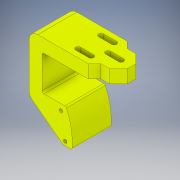
# Autodesk Inventor part: holder_outer
Saved by Autodesk Inventor 2019 (Build 230136000, 136)
## iProperties
Created: 2019-01-30
Part Number: holder_outer
Material: Generic
Document SubType Name: Modeling
Designer: suchanek
Density: 1 g/cm^3
Appearance: Default
Author: suchanek
Autodesk Inventor part; units mm, degrees
ref_plane "YZ Plane" through (0, 0, 0) normal (1, 0, 0) x (0, 1, 0)
ref_plane "XZ Plane" through (0, 0, 0) normal (0, 1, 0) x (-1, 0, 0)
ref_plane "XY Plane" through (0, 0, 0) normal (0, 0, 1) x (1, 0, 0)
sketch "Sketch1" plane through (0, 0, 0) normal (0, 0, 1) x (1, 0, 0)
  line L0 (-10, 0) -> (0, 0)
  line L1 (0, 0) -> (17.3648, -98.4808)
  line L2 (17.3648, -98.4808) -> (27.2129, -96.7443)
  line L3 (27.2129, -96.7443) -> (8.391, 10)
  line L4 (8.391, 10) -> (-10, 10)
  line L5 (-10, 10) -> (-10, 0)
  dimension "d0" = 80
  dimension "d1" = 10
  dimension "d2" = 10
  dimension "d3" = 10
  dimension "d4" = 100
  constraints: 12 end point, 4 perpendicular, 1 horizontal
  measures "d0" angle of L0 L1
  measures "d1" distance of L0.start L0.end
  measures "d2" distance between parallel lines of L4 L0
  measures "d3" distance between parallel lines of L1 L3
  measures "d4" distance of L0.end L1.end
sketch "Sketch2" plane through (0, 0, 0) normal (0, 0, 1) x (1, 0, 0)
  line L0 (18.1173, -67.6148) -> (56.6427, 18.898)
  line L1 (27.94, 25) -> (-20, 10)
  line L2 (0, 0) -> (-20, 0)
  line L3 (-20, 0) -> (-20, 10)
  line L4 (0, 0) -> (18.1173, -67.6148)
  line L5 (0, 0) -> (70, 0) construction
  circle A0 centre (42.94, 25) radius 15
  circle A1 centre (42.94, 25) radius 5
  line L6 (-20, 10) -> (25, 10)
  dimension "d5" = 20
  dimension "d6" = 10
  dimension "d7" = 70
  dimension "d8" = 75
  dimension "d9" = 30
  dimension "d10" = 10
  dimension "d61" = 62.94
  constraints: 14 end point, 3 horizontal, 2 centre point, 2 point on circle, 2 tangent, 1 coincident, 1 equal length, 1 horizontal alignment, 1 vertical
  measures "d5" distance of L2.start L2.end
  measures "d6" distance of L2.end L1.end
  measures "d7" distance of L2.start L0.start
  measures "d8" angle of L4 L5
  measures "d9" diameter of A0
  measures "d10" diameter of A1
  measures "d61" distance from line of A0.centre L3
extrude "Extrusion1" add sketch "Sketch1" along normal mid plane 100
extrude "Extrusion2" add sketch "Sketch2" along normal mid plane 30
sketch "Sketch3" plane through (0, 0, 15) normal (0, 0, 1) x (1, 0, 0)
  line L0 (20.9536, -61.2458) -> (8.391, 10) projected
  line L1 (56.6427, 10) -> (8.391, 10)
  arc A0 (56.6427, 18.898) -> (27.94, 25) centre (42.94, 25) ccw projected
  line L2 (57.94, 25) -> (57.94, -20)
  line L3 (57.94, -20) -> (13.6808, -20)
  line L4 (20.9536, -61.2458) -> (56.6427, 18.898) projected
  line L5 (56.6427, 10) -> (57.94, 10)
  point P0 (42.941, 25)
  point P1 (9.2838, 4.9367)
  point P2 (57.94, 10)
  dimension "d23" = 30
  constraints: 8 end point, 3 point on line, 2 perpendicular, 1 horizontal, 1 point on circle, 1 tangent, 1 vertical
  measures "d23" distance between parallel lines of L3 L1
extrude "Extrusion3" add sketch "Sketch3" against normal up to surface (100 mm away) from surface at 35 contours L0 L1 L4 L3 | L4 L1 L5 L2 L3 | L4 A0 L2 L5 L1
extrude "Extrusion5" add sketch "Sketch3" against normal up to surface (30 mm away)
sketch "Sketch5" plane through (57.94, 10, 15) normal (1, 0, 0) x (0, 0, -1)
  line L0 (65, -10) -> (-35, -10) projected
  line L1 (-23, -10) -> (-3, -10)
  line L2 (-3, -10) -> (-3, -20)
  line L3 (-3, -20) -> (-23, -20)
  line L4 (-23, -20) -> (-23, -10)
  line L5 (0, 0) -> (0, 15) projected
  line L6 (15, -10) -> (15, 0)
  line L7 (53, -10) -> (33, -10)
  line L8 (33, -10) -> (33, -20)
  line L9 (33, -20) -> (53, -20)
  line L10 (53, -20) -> (53, -10)
  dimension "d26" = 20
  dimension "d27" = 10
  dimension "d28" = 3
  constraints: 18 end point, 4 symmetric about line, 2 parallel, 1 horizontal, 1 perpendicular, 1 point on line, 1 vertical
  measures "d26" distance of L2.end L3.end
  measures "d27" distance of L1.end L2.end
  measures "d28" distance between parallel lines of L5 L2
extrude "Extrusion6" cut sketch "Sketch5" against normal blind 50
sketch "Sketch6" plane through (-10, 10, 50) normal (0, 1, 0) x (1, 0, 0)
  circle A0 centre (32.94, 22) radius 2.6
  line L0 (32.94, 22) -> (54.1621, 22)
  line L1 (67.94, 32) -> (17.94, 32) projected
  line L2 (67.94, 32) -> (72.1451, 32)
  line L3 (67.94, 12) -> (17.94, 12) projected
  line L4 (67.94, 12) -> (72.1451, 12)
  line L5 (67.94, 32) -> (70.0688, 32)
  line L6 (67.94, 12) -> (80.0698, 12)
  arc A1 (56.4323, 13.4495) -> (56.4323, 30.5505) centre (32.94, 22) ccw
  line L7 (32.94, 22) -> (56.4323, 13.4495) construction
  line L8 (32.94, 22) -> (57.94, 22) construction
  line L9 (32.94, 22) -> (56.4323, 30.5505) construction
  arc A2 (61.3187, 11.671) -> (61.3187, 32.329) centre (32.94, 22) ccw
  line L10 (32.94, 22) -> (61.3187, 11.671) construction
  line L11 (32.94, 22) -> (63.14, 22) construction
  line L12 (32.94, 22) -> (61.3187, 32.329) construction
  arc A3 (61.3187, 32.329) -> (56.4323, 30.5505) centre (58.8755, 31.4398) ccw
  arc A4 (56.4323, 13.4495) -> (61.3187, 11.671) centre (58.8755, 12.5602) ccw
  line L13 (67.94, 35) -> (67.94, 0) projected
  point P0 (10, 50)
  point P1 (77.941, 35)
  point P2 (77.941, 5)
  point P3 (77.941, 0)
  dimension "d31" = 5.2
  dimension "d35" = 25
  dimension "d36" = 20
  dimension "d37" = 40
  dimension "d38" = 30.2
  dimension "d39" = 20
  dimension "d40" = 40
  dimension "d41" = 35
  constraints: 22 end point, 12 point on circle, 5 centre point, 5 horizontal, 3 coincident, 2 equal length, 2 point on line, 2 tangent, 2 other
  measures "d31" diameter of A0
  measures "d35" radius of A1
  measures "d36" angle of L7 L8
  measures "d37" angle of L7 L9
  measures "d38" radius of A2
  measures "d39" angle of L10 L11
  measures "d40" angle of L10 L12
extrude "Extrusion7" cut sketch "Sketch6" against normal up to surface (30 mm away) contours A0 | A2 L3 A4 A1 A3 L1 | L1 A3 A2 | A2 A4 L3
sketch "Sketch8" plane through (-10, 10, 50) normal (0, 1, 0) x (1, 0, 0)
  circle A0 centre (68.8765, 31.4398) radius 4.6
  arc A1 (71.3197, 32.329) -> (66.4333, 30.5505) centre (68.8765, 31.4398) ccw projected
  point P0 (10, 50)
  dimension "d49" = 9.2
  constraints: 1 centre point, 1 concentric
  measures "d49" diameter of A0
extrude "Extrusion9" cut sketch "Sketch8" along normal through all
sketch "Sketch9" plane through (57.94, 10, 15) normal (1, 0, 0) x (0, 0, -1)
  line L0 (-31, -20) -> (5, -20)
  line L1 (5, -20) -> (5, -10)
  line L2 (5, -10) -> (-31, -10)
  line L3 (-31, -10) -> (-31, -20)
  line L4 (-3, -20) -> (-23, -20) projected
  line L5 (-23, -10) -> (-3, -10) projected
  line L6 (-3, -10) -> (-3, -20) projected
  line L7 (-23, -20) -> (-23, -10) projected
  point P0 (15, -10)
  dimension "d53" = 8
  dimension "d58" = 8
  constraints: 8 end point, 2 collinear, 2 parallel, 1 horizontal, 1 perpendicular
  measures "d53" distance between parallel lines of L1 L6
  measures "d58" distance between parallel lines of L7 L3
loft "Loft1" cut profiles "Sketch9" section 2 edges at (7.94, -5, 38) (7.94, -10, 28) (7.94, -5, 18) (7.94, 0, 28)
mirror "Mirror2" about plane through (0, 0, 0) normal (0, 0, 1) of "Extrusion7", "Extrusion9", "Loft1"
sketch "Sketch10" plane through (0, 0, -15) normal (0, 0, -1) x (-1, 0, 0)
  line L0 (-57.941, 10) -> (10, 10)
  line L1 (10, 10) -> (10, 40)
  line L2 (10, 40) -> (-57.941, 40)
  line L3 (-57.941, 40) -> (-57.941, 10)
  arc A0 (-27.94, 25) -> (-55.9636, 32.4421) centre (-42.94, 25) ccw projected
  point P0 (0, 0)
  constraints: 8 end point, 2 parallel, 1 horizontal, 1 perpendicular, 1 point on line, 1 tangent
extrude "Extrusion10" cut sketch "Sketch10" along normal through all both and the other way through all
sketch "Sketch11" plane through (13.6808, -20, 15) normal (0, -1, 0) x (1, 0, 0)
  circle A0 centre (9.2592, 13) radius 2.6 projected
  line L0 (6.8632, 8.85) -> (4.4672, 13)
  line L1 (4.4672, 13) -> (6.8632, 17.15)
  line L2 (6.8632, 17.15) -> (11.6552, 17.15)
  line L3 (11.6552, 17.15) -> (14.0512, 13)
  line L4 (14.0512, 13) -> (11.6552, 8.85)
  line L5 (11.6552, 8.85) -> (6.8632, 8.85)
  circle A1 centre (9.2592, -43) radius 2.6 projected
  line L6 (6.8632, -47.15) -> (4.4672, -43)
  line L7 (4.4672, -43) -> (6.8632, -38.85)
  line L8 (6.8632, -38.85) -> (11.6552, -38.85)
  line L9 (11.6552, -38.85) -> (14.0512, -43)
  line L10 (14.0512, -43) -> (11.6552, -47.15)
  line L11 (11.6552, -47.15) -> (6.8632, -47.15)
  point P0 (-13.6808, -15)
  point P1 (9.2592, 13)
  point P2 (9.2592, -43)
  point P3 (9.2592, 8.85)
  dimension "d62" = 8.3
  dimension "d63" = 8.3
  constraints: 24 end point, 2 coincident, 1 horizontal, 1 horizontal alignment, 1 midpoint, 26 other
  measures "d62" distance between parallel lines of L10 L7
  measures "d63" distance between parallel lines of L5 L2
extrude "Extrusion11" cut sketch "Sketch11" against normal blind 3
sketch "Sketch12" plane through (-10, 0, 50) normal (0, -1, 0) x (1, 0, 0)
  line L0 (14.396, -41) -> (12, -36.85)
  line L1 (12, -36.85) -> (14.396, -32.7)
  line L2 (14.396, -32.7) -> (19.188, -32.7)
  line L3 (19.188, -32.7) -> (21.584, -36.85)
  line L4 (21.584, -36.85) -> (19.188, -41)
  line L5 (19.188, -41) -> (14.396, -41)
  line L6 (19.188, -59) -> (21.584, -63.15)
  line L7 (21.584, -63.15) -> (19.188, -67.3)
  line L8 (19.188, -67.3) -> (14.396, -67.3)
  line L9 (14.396, -67.3) -> (12, -63.15)
  line L10 (12, -63.15) -> (14.396, -59)
  line L11 (14.396, -59) -> (19.188, -59)
  line L12 (10, -50) -> (9.9797, -50)
  line L13 (10, -100) -> (10, 0) projected
  line L14 (10, -54.6091) -> (9.2997, -54.6091)
  line L15 (14.396, -67.3) -> (14.396, -59)
  line L16 (14.396, -41) -> (14.396, -32.7)
  line L17 (14.396, -41) -> (10, -41)
  line L18 (10, -41) -> (10, -32.7)
  line L19 (10, -32.7) -> (14.396, -32.7)
  line L20 (14.396, -32.7) -> (14.396, -41)
  line L21 (14.396, -67.3) -> (10, -67.3)
  line L22 (10, -67.3) -> (10, -59)
  line L23 (10, -59) -> (14.396, -59)
  line L24 (14.396, -59) -> (14.396, -67.3)
  circle A0 centre (16.792, -63.15) radius 2.8
  circle A1 centre (16.792, -36.85) radius 2.8
  dimension "d66" = 8.3
  dimension "d67" = 8.3
  dimension "d68" = 9
  dimension "d99" = 2
  dimension "d102" = 5.6
  dimension "d103" = 5.6
  constraints: 48 end point, 4 horizontal, 4 parallel, 3 collinear, 3 vertical, 2 centre point, 2 coincident, 2 perpendicular, 1 point on line, 32 other
  measures "d66" distance between parallel lines of L11 L8
  measures "d67" distance between parallel lines of L2 L5
  measures "d68" distance between parallel lines of L12 L11
  measures "d102" diameter of A0
  measures "d103" diameter of A1
extrude "Extrusion12" cut sketch "Sketch12" along normal blind 6 contours L16 A1 L2 L3 L4 L5 | L0 L1 L16 A1 | A1 L16 | L16 A1 | L6 L7 L8 L15 A0 L11 | L15 A0 L9 L10 | A0 L15 | L15 A0
extrude "Extrusion15" cut sketch "Sketch12" along normal blind 6 contours L17 L13 L19 L1 L0 | L16 A1 L2 L3 L4 L5 | L16 A1 | L6 L7 L8 L15 A0 L11 | L15 A0 L9 L10 | L10 L9 L21 L13 L23 | A0 L15 | L15 A0 picked at (16.128, -36.85)
sketch "Sketch15" plane through (0, 0, 15) normal (0, 0, 1) x (1, 0, 0)
  line L0 (-20, 0) -> (-20, 10) projected
  line L1 (-10, 13.1289) -> (-20, 10) projected
  line L2 (-20, 0) -> (-10, 0)
  line L3 (-10, 0) -> (-10, 13.1289)
  line L4 (-10, 13.1289) -> (-20, 13.1289)
  line L5 (-20, 13.1289) -> (-20, 0)
  point P0 (0, 0)
  constraints: 8 end point, 2 parallel, 1 horizontal, 1 perpendicular
extrude "Extrusion17" cut sketch "Sketch15" against normal blind 100 contours L0 L1 L3 L2
sketch "Sketch17" plane through (-10, 10, 50) normal (0, 1, 0) x (1, 0, 0)
  line L0 (0, 0) -> (0, 100) projected
  line L1 (27.3648, 0) -> (27.3648, 100) projected
  line L2 (0, 72.2615) -> (27.3648, 72.2615)
  line L3 (27.3648, 72.2615) -> (27.3648, 27.7385)
  line L4 (27.3648, 27.7385) -> (0, 27.7385)
  line L5 (0, 27.7385) -> (0, 72.2615)
  circle A0 centre (32.94, 78) radius 2.6 projected
  circle A1 centre (32.94, 22) radius 2.6 projected
  line L6 (27.3648, 27.7385) -> (34.6263, 35)
  line L7 (34.6263, 35) -> (44.6263, 35)
  line L8 (44.6263, 35) -> (54.6263, 45)
  line L9 (54.6263, 45) -> (54.6263, 55)
  line L10 (54.6263, 55) -> (44.6263, 65)
  line L11 (44.6263, 65) -> (34.6263, 65)
  line L12 (34.6263, 65) -> (27.3648, 72.2615)
  point P0 (10, 50)
  dimension "d134" = 8
  dimension "d135" = 8
  dimension "d136" = 45
  dimension "d137" = 45
  dimension "d138" = 135
  dimension "d139" = 135
  dimension "d140" = 10
  dimension "d141" = 30
  constraints: 22 end point, 3 horizontal, 3 point on line, 2 equal length, 2 parallel, 1 perpendicular, 1 vertical
  measures "d134" distance from line of A0.centre L12
  measures "d135" distance from line of A1.centre L6
  measures "d136" angle of L3 L6
  measures "d137" angle of L3 L12
  measures "d138" angle of L11 L10
  measures "d139" angle of L8 L7
  measures "d140" distance of L8.end L9.end
  measures "d141" distance between parallel lines of L11 L7
extrude "Extrusion18" add sketch "Sketch17" along normal blind 15 contours L0 L2 L1 L4 | L1 L12 L11 L10 L9 L8 L7 L6
extrude "Extrusion16" cut sketch "Sketch12" against normal blind 100 and the other way blind 10 contours A1 L16 | L16 A1 | A0 L15 | L15 A0
sketch "Sketch13" plane through (-10, 10, 50) normal (0, 1, 0) x (1, 0, 0)
  line L0 (10, 50) -> (37.94, 50)
  line L1 (27.3648, 0) -> (27.3648, 100) projected
  circle A0 centre (37.94, 50) radius 2.8
  line L2 (67.94, 100) -> (67.94, 0) projected
  dimension "d85" = 5.6
  dimension "d108" = 30
  constraints: 2 end point, 1 centre point, 1 coincident, 1 horizontal
  measures "d85" diameter of A0
  measures "d108" distance from line of A0.centre L2
extrude "Extrusion13" cut sketch "Sketch13" against normal blind 30 and the other way blind 150
sketch "Sketch14" plane through (27.94, -20, 0) normal (0, 1, 0) x (1, 0, 0)
  line L0 (-10.5752, -50) -> (-10.5752, 50) projected
  line L1 (-2.4249, -4.2) -> (-4.8497, 0)
  line L2 (-4.8497, 0) -> (-2.4249, 4.2)
  line L3 (-2.4249, 4.2) -> (2.4249, 4.2)
  line L4 (2.4249, 4.2) -> (4.8497, 0)
  line L5 (4.8497, 0) -> (2.4249, -4.2)
  line L6 (2.4249, -4.2) -> (-2.4249, -4.2)
  circle A0 centre (0, 0) radius 2.8 projected
  line L7 (-2.4249, 4.2) -> (-32.4249, 4.2)
  line L8 (-32.4249, 4.2) -> (-32.4249, -4.2)
  line L9 (-32.4249, -4.2) -> (-2.4249, -4.2)
  line L10 (-2.4249, -4.2) -> (-2.4249, 4.2)
  point P0 (-27.94, 0)
  point P1 (-10.5752, -4.2)
  dimension "d88" = 8.4
  dimension "d89" = 30
  constraints: 20 end point, 2 coincident, 2 horizontal, 2 parallel, 1 collinear, 1 perpendicular, 1 point on line, 15 other
  measures "d88" distance between parallel lines of L3 L6
  measures "d89" distance of L2.end L7.end
hole "Hole3" at (27.94, -20, 0) direction (0, -1, 0) diameter 5.2 depth 5 tip angle 118
extrude "Extrusion14" cut sketch "Sketch14" along normal blind 6
sketch "Sketch18" plane through (-10, 10, 22.2615) normal (0, 0, 1) x (1, 0, 0)
  line L0 (0, 0) -> (0, 15) projected
  line L1 (0, 0) -> (-25, 0)
  line L2 (-25, 0) -> (-25, -40)
  line L3 (-25, -40) -> (2.0893, -40)
  line L4 (9.0352, -79.3923) -> (-0.9648, -79.3923)
  line L5 (-0.9648, -79.3923) -> (-40, -50)
  line L6 (-40, -50) -> (-40, 15)
  line L7 (0, 15) -> (27.3648, 15) projected
  line L8 (-40, 15) -> (0, 15)
  line L9 (0, 0) -> (0, -10) projected
  line L10 (0, -10) -> (10, -10) projected
  line L11 (10, -10) -> (27.3648, -108.4808) projected
  arc A0 (9.0352, -79.3923) -> (2.0893, -40) centre (-67.9448, -72.6574) ccw
  line L12 (2.0893, -40) -> (9.0352, -79.3923)
  dimension "d120" = 25
  dimension "d125" = 10
  dimension "d126" = 15
  dimension "d127" = 10
  dimension "d128" = 40
  dimension "d149" = 30
  dimension "d150" = 13
  dimension "d158" = 40
  constraints: 16 end point, 3 perpendicular, 2 horizontal, 2 parallel, 2 point on circle, 1 centre point
  measures "d120" distance between parallel lines of L9 L2
  measures "d125" distance of L4.start L4.end
  measures "d126" distance between parallel lines of L2 L6
  measures "d127" distance from line of L5.end L3
  measures "d128" distance of L3.end L4.start
  measures "d150" distance between parallel lines of L11 L12
  measures "d158" distance of L1.end L2.end
extrude "Extrusion19" add sketch "Sketch18" against normal up to surface (44.5229 mm away)
sketch "Sketch19" plane through (-10, 25, 50) normal (0, 1, 0) x (1, 0, 0)
  line L0 (21.792, 63.15) -> (6.792, 63.15) construction
  line L1 (21.792, 65.95) -> (6.792, 65.95)
  line L2 (6.792, 60.35) -> (21.792, 60.35)
  arc A0 (21.792, 60.35) -> (21.792, 65.95) centre (21.792, 63.15) ccw
  arc A1 (6.792, 65.95) -> (6.792, 60.35) centre (6.792, 63.15) ccw
  line L3 (10, 50) -> (16.7162, 50)
  circle A2 centre (16.792, 63.15) radius 2.8 projected
  line L4 (21.792, 36.85) -> (6.792, 36.85) construction
  line L5 (21.792, 34.05) -> (6.792, 34.05)
  line L6 (6.792, 39.65) -> (21.792, 39.65)
  arc A3 (21.792, 34.05) -> (21.792, 39.65) centre (21.792, 36.85) ccw
  arc A4 (6.792, 39.65) -> (6.792, 34.05) centre (6.792, 36.85) ccw
  circle A5 centre (37.94, 50) radius 2.8 projected
  line L7 (42.94, 50) -> (27.94, 50) construction
  line L8 (42.94, 52.8) -> (27.94, 52.8)
  line L9 (27.94, 47.2) -> (42.94, 47.2)
  arc A6 (42.94, 47.2) -> (42.94, 52.8) centre (42.94, 50) ccw
  arc A7 (27.94, 52.8) -> (27.94, 47.2) centre (27.94, 50) ccw
  point P0 (14.292, 63.15)
  point P1 (14.292, 36.85)
  point P2 (16.792, 36.85)
  point P3 (35.44, 50)
  dimension "d131" = 10
  dimension "d132" = 5
  dimension "d133" = 5
  constraints: 26 end point, 12 point on circle, 9 tangent, 8 symmetric about line, 6 centre point, 3 horizontal, 3 parallel, 2 equal radius, 2 midpoint, 1 coincident, 1 horizontal alignment, 2 other
  measures "d131" distance of A2.centre L0.end
  measures "d132" distance of A2.centre L0.start
  measures "d133" distance of L7.start A5.centre
extrude "Extrusion20" cut sketch "Sketch19" against normal blind 15 contours A0 L2 A2 L1 | A2 L2 A1 L1 | L5 A4 L6 A3 | A5 L8 A6 L9 | A5 L9 A7 L8
sketch "Sketch20" plane through (0, 0, 50) normal (0, 0, 1) x (1, 0, 0)
  line L0 (-10, 10) -> (-10, 0) projected
  line L1 (57.94, 10) -> (57.94, -20) projected
  line L2 (-10, 10) -> (57.94, 10)
  line L3 (57.94, 10) -> (57.94, -20)
  line L4 (13.6808, -20) -> (27.2129, -96.7443) projected
  line L5 (57.94, -20) -> (27.2129, -96.7443)
  line L6 (17.3648, -98.4808) -> (0, 0) projected
  line L7 (27.2129, -96.7443) -> (17.3648, -98.4808)
  line L8 (17.3648, -98.4808) -> (0, 0)
  line L9 (0, 0) -> (-10, 0) projected
  line L10 (0, 0) -> (-10, 0)
  line L11 (-10, 0) -> (-10, 10)
  constraints: 14 end point, 3 collinear, 3 perpendicular
extrude "Extrusion21" cut sketch "Sketch20" along normal through all both and the other way through all
fillet "Fillet1" radius 10 3 edges at (-50, 25, 0) (-50, -40, 0) (-10.9648, -69.3923, 0)
fillet "Fillet2" radius 2 4 edges at (-35, -30, 0) (-7.9107, -30, 0) (-0.9648, -69.3923, 0) (-35, 10, 0)
sketch "Sketch21" plane through (17.3648, 10, 22.2615) normal (0, 0, 1) x (1, 0, 0)
  circle A0 centre (-30.9622, -47) radius 2
  circle A1 centre (-26.0698, -74.835) radius 2
  arc A2 (-26.0698, -74.835) -> (-30.9622, -47) centre (-95.3096, -72.6574) ccw
  arc A3 (-18.1886, -77.5181) -> (-24.7349, -41.1854) centre (-95.3096, -72.6574) ccw projected
  line L0 (-63.38, -53.0005) -> (-31.0009, -77.3809) projected
  line L1 (-26.5615, -40) -> (-50.3648, -40) projected
  point P0 (-17.3648, -10)
  dimension "d151" = 4
  dimension "d152" = 4
  dimension "d153" = 8
  dimension "d154" = 5
  dimension "d155" = 7
  constraints: 3 centre point, 2 point on circle, 1 concentric
  measures "d151" diameter of A0
  measures "d152" diameter of A1
  measures "d153" radial gap between concentric circles of A3 A2
  measures "d154" distance from line of L0 A1.centre
  measures "d155" distance from line of L1 A0.centre
extrude "Extrusion22" cut sketch "Sketch21" against normal blind 5
mirror "Mirror3" about plane through (0, 0, 0) normal (0, 0, 1) of "Extrusion22"
equation "\"d0\" = boat_rim_angle"
equation "\"d3\" = d2"
equation "\"boat_rim_angle\" = 80deg"
body "Solid1"
